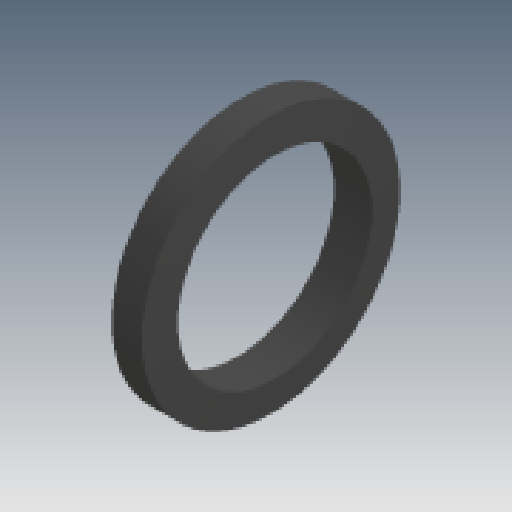
# Autodesk Inventor part: 低速轴油封
Saved by Autodesk Inventor 2025 (Build 290162000, 162)
## iProperties
Created: 2025-03-19
Part Number: 低速轴油封
Material: 橡胶
Document SubType Name: Modeling
Designer: liukan
Density: 0.93 g/cm^3
Appearance: 橡胶 - 黑色
Author: liukan
Autodesk Inventor part; units mm, degrees
ref_plane "YZ Plane" through (0, 0, 0) normal (1, 0, 0) x (0, 1, 0)
ref_plane "XZ Plane" through (0, 0, 0) normal (0, 1, 0) x (-1, 0, 0)
ref_plane "XY Plane" through (0, 0, 0) normal (0, 0, 1) x (1, 0, 0)
sketch "草图1" plane through (0, 0, 0) normal (0, 0, 1) x (1, 0, 0)
  line L0 (-4, -30) -> (-3.1405, -23)
  line L1 (-4, -30) -> (-11, -30) projected
  line L2 (-11, -30) -> (-11.8595, -23) projected
  line L3 (-11, -30) -> (-4, -30)
  line L4 (-11, -30) -> (-11.8595, -23) projected
  line L5 (-11, -30) -> (-11.8595, -23) projected
  line L6 (-11, -30) -> (-11.8595, -23) projected
  line L7 (-11, -30) -> (-11.8595, -23) projected
  line L8 (-12, 65) -> (-12, -65) projected
  line L9 (-11, -30) -> (-11.8595, -23) projected
  line L10 (0, 0) -> (-15, 0) construction
  line L11 (-11, -30) -> (-11.8595, -23) projected
  line L12 (-11.8595, -23) -> (-11, -30)
  line L13 (-11.8595, -23) -> (-11, -30)
  line L14 (-11.8595, -23) -> (-11, -30)
  line L15 (-4, -30) -> (-3.0791, -22.5)
  line L16 (-3.0791, -22.5) -> (-11.9209, -22.5)
  line L17 (-11.9209, -22.5) -> (-11, -30)
  dimension "d0" = 22.5
  constraints: 16 end point, 2 collinear, 1 horizontal, 1 perpendicular, 6 other
  measures "d0" distance between parallel lines of L10 L16
revolve "旋转1" add sketch "草图1" angle 360 about axis through (0, 0, 0) along (-1, 0, 0)
